Tray spacers  better (Autodesk Fusion 360 archive; units mm, degrees)
design "tray spacers"
Autodesk Fusion 360 part; units mm, degrees
(part 1 of 2)
sketch "Sketch1" plane through (0, 0, 0) normal (0, 1, 0) x (1, 0, 0)
  line L0 (21, -7) -> (-21, -7)
  line L1 (-21, -7) -> (-21, 7)
  line L2 (-21, 7) -> (21, 7)
  line L3 (21, 7) -> (21, -7)
  line L4 (21, -7) -> (-21, 7) construction
  line L5 (-21, -7) -> (21, 7) construction
  line L6 (7, -21) -> (-7, -21)
  line L7 (-7, -21) -> (-7, 21)
  line L8 (-7, 21) -> (7, 21)
  line L9 (7, 21) -> (7, -21)
  line L10 (7, -21) -> (-7, 21) construction
  line L11 (-7, -21) -> (7, 21) construction
  line L12 (23.58, 0) -> (93.58, 0)
  line L13 (93.58, 0) -> (93.58, 7)
  line L14 (93.58, 7) -> (23.58, 7)
  line L15 (23.58, 7) -> (23.58, 0)
  line L16 (58.58, 0) -> (51.58, 0)
  line L17 (51.58, 0) -> (51.58, 42)
  line L18 (51.58, 42) -> (58.58, 42)
  line L19 (58.58, 42) -> (58.58, 0)
  line L20 (58.58, 0) -> (65.58, 0)
  line L21 (65.58, 0) -> (65.58, 42)
  line L22 (65.58, 42) -> (58.58, 42)
  line L23 (58.58, 42) -> (58.58, 0)
  line L24 (101.6, 0) -> (143.6, 0)
  line L25 (143.6, 0) -> (143.6, 7)
  line L26 (143.6, 7) -> (101.6, 7)
  line L27 (101.6, 7) -> (101.6, 0)
  line L28 (143.6, 0) -> (136.6, 0)
  line L29 (136.6, 0) -> (136.6, 42)
  line L30 (136.6, 42) -> (143.6, 42)
  line L31 (143.6, 42) -> (143.6, 0)
  line L32 (-21, 57) -> (21, 57)
  line L33 (7, 71) -> (7, 29)
  line L34 (21, 57) -> (21, 43)
  line L35 (21, 43) -> (-21, 57) construction
  line L36 (-21, 43) -> (21, 57) construction
  line L37 (-7, 29) -> (7, 71) construction
  line L38 (21, 43) -> (-21, 43)
  line L39 (-21, 43) -> (-21, 57)
  line L40 (-7, 29) -> (-7, 71)
  line L41 (7, 29) -> (-7, 71) construction
  line L42 (-7, 71) -> (7, 71)
  line L43 (7, 29) -> (-7, 29)
  line L44 (93.58, 0) -> (23.58, 0)
  line L45 (23.58, 0) -> (23.58, -7)
  line L46 (23.58, -7) -> (93.58, -7)
  line L47 (93.58, -7) -> (93.58, 0)
  line L48 (101.6, 0) -> (150.6, 0)
  line L49 (150.6, 0) -> (150.6, -7)
  line L50 (150.6, -7) -> (101.6, -7)
  line L51 (101.6, -7) -> (101.6, 0)
  line L52 (150.6, -7) -> (143.6, -7)
  line L53 (143.6, -7) -> (143.6, 42)
  line L54 (143.6, 42) -> (150.6, 42)
  line L55 (150.6, 42) -> (150.6, -7)
  point P0 (0, 50)
  point P1 (0, 50)
  dimension "d1" = 42
  dimension "d2" = 14
  dimension "d3" = 14
  dimension "d4" = 42
  dimension "d5" = 70
  dimension "d6" = 7
  dimension "d7" = 7
  dimension "d8" = 42
  dimension "d9" = 7
  dimension "d10" = 42
  dimension "d11" = 42
  dimension "d12" = 7
  dimension "d13" = 7
  dimension "d14" = 42
  dimension "d15" = 42
  dimension "d16" = 14
  dimension "d17" = 14
  dimension "d18" = 42
  dimension "d25" = 7
  dimension "d26" = 49
  dimension "d27" = 7
  constraint horizontal L0
  constraint perpendicular L0 L1
  constraint parallel L0 L2
  constraint parallel L1 L3
  constraint coincident L4 origin
  constraint coincident L5 origin
  constraint horizontal L6
  constraint perpendicular L6 L7
  constraint parallel L6 L8
  constraint parallel L7 L9
  constraint coincident L10 origin
  constraint coincident L11 origin
  constraint horizontal L12
  constraint vertical L13
  constraint horizontal L14
  constraint vertical L15
  constraint horizontal L16
  constraint vertical L17
  constraint horizontal L18
  constraint vertical L19
  constraint midpoint L12 L16.start
  constraint horizontal L20
  constraint vertical L21
  constraint horizontal L22
  constraint vertical L23
  constraint horizontal L24
  constraint vertical L25
  constraint horizontal L26
  constraint vertical L27
  constraint horizontal L28
  constraint vertical L29
  constraint horizontal L30
  constraint vertical L31
  constraint horizontal L38
  constraint perpendicular L38 L39
  constraint parallel L32 L38
  constraint parallel L34 L39
  constraint coincident P1 L35
  constraint coincident P1 L36
  constraint horizontal L43
  constraint perpendicular L40 L43
  constraint parallel L42 L43
  constraint parallel L33 L40
  constraint coincident P1 L41
  constraint coincident P1 L37
  constraint coincident P1 P0
  constraint horizontal L44
  constraint vertical L45
  constraint horizontal L46
  constraint vertical L47
  constraint horizontal L48
  constraint vertical L49
  constraint horizontal L50
  constraint vertical L51
  constraint horizontal L52
  constraint vertical L53
  constraint horizontal L54
  constraint vertical L55
  measures "d1" distance of L1.end L2.end
  measures "d2" distance of L0.end L1.end
  measures "d3" distance of L7.end L8.end
  measures "d4" distance of L6.end L7.end
  measures "d5" distance of L12.start L12.end
  measures "d6" distance of L12.start L14.end
  measures "d7" distance of L16.start L16.end
  measures "d8" distance of L16.start L18.end
  measures "d9" distance of L16.start L20.end
  measures "d10" distance of L16.start L18.end
  measures "d11" distance of L24.start L24.end
  measures "d12" distance of L24.start L26.end
  measures "d13" distance of L24.end L28.end
  measures "d14" distance of L24.end L30.end
  measures "d15" distance of L32.start L32.end
  measures "d16" distance of L36.start L32.start
  measures "d17" distance of L33.start L40.end
  measures "d18" distance of L40.end L37.start
  measures "d25" distance of L12.end L46.end
  measures "d26" distance of L24.start L48.end
  measures "d27" distance of L24.start L50.end
extrude "Extrude1" add sketch "Sketch1" along normal blind 54 contours L0 L2 L3 L9 | L0 L6 L7 L9 | L0 L2 L7 L9 | L0 L1 L2 L7 | L2 L7 L8 L9 | L12 L14 L15 L17 L44 | L12 L16 L20 L44 L45 L46 L47 | L12 L14 L16 L17 L19 L23 L44 | L12 L14 L19 L20 L21 L23 L44 | L14 L17 L18 L19 L23 | L12 L13 L14 L21 L44 | L14 L19 L21 L22 L23 | L24 L26 L27 L29 L48 | L24 L28 L48 L50 L51 L53 | L24 L25 L26 L28 L29 L31 L48 L53 | L25 L31 L48 L53 L54 L55 | L48 L49 L50 L52 L53 L55 | L26 L29 L30 L31 L53 makes body 1 at (-16.3333, 0, -2.3333) makes body 2 at (46.9133, 18, 7) makes body 3 at (134.2667, 36, 7)
extrude "Extrude2" add sketch "Sketch1" along normal blind 12 separate body contours L32 L38 L39 L40 | L32 L33 L40 L42 | L32 L33 L38 L40 | L32 L33 L34 L38 | L33 L38 L40 L43 makes body 4
chamfer "Chamfer1" distance 6.99 angle 59 7 edges at (79.58, 54, -7) (65.58, 54, -24.5) (58.58, 54, -42) (51.58, 54, -24.5) (37.58, 54, -7) (136.6, 54, -24.5) (119.1, 54, -7) 2 faces at (-16.3333, 54, -2.3333) (-2.3333, 12, -33.6667) measured on face at (56.2467, 54, 2.3333) measured on face at (56.2467, 54, 2.3333) measured on face at (56.2467, 54, 2.3333) measured on face at (56.2467, 54, 2.3333) measured on face at (56.2467, 54, 2.3333) measured on face at (129.6, 54, 2.3333) measured on face at (129.6, 54, 2.3333) tangent chain off on bodies 1 2 3 4
extrude "Extrude3" add 2 faces at (131.93, 54, 4.6633) (58.5767, 54, 4.6633) along direction (0, 1, 0) blind 3 on bodies 2 3 bodies 3 2
extrude "Extrude4" cut 1 faces at (58.57, 55, -11.6767) along direction (1, 0, 0) blind 1 on bodies 2 bodies 2
sketch "Sketch2" plane through (0, 0, 7) normal (0, 0, 1) x (1, 0, 0)
  line L0 (23.58, 0) -> (93.58, 0)
  line L1 (93.58, 0) -> (93.58, 57)
  line L2 (93.58, 57) -> (23.58, 57)
  line L3 (23.58, 57) -> (23.58, 0)
  line L4 (93.58, 0) -> (58.58, 0)
  line L5 (58.58, 0) -> (58.58, 12)
  line L6 (58.58, 12) -> (93.58, 12)
  line L7 (93.58, 12) -> (93.58, 0)
  line L8 (58.58, 12) -> (58.58, 45)
  circle A0 centre (58.58, 12) radius 1.9
  circle A1 centre (58.58, 45) radius 1.9
  dimension "d32" = 35
  dimension "d33" = 12
  dimension "d34" = 33
  dimension "d35" = 3.8
  dimension "d36" = 3.8
  constraint horizontal L4
  constraint vertical L5
  constraint horizontal L6
  constraint vertical L7
  constraint coincident L0.end L1.start
  constraint perpendicular L6 L8
  constraint coincident L5.end L6.start
  constraint coincident L8.end A1.centre
  measures "d32" distance of L0.end L4.end
  measures "d33" distance of L0.end L6.end
  measures "d34" distance of L5.end L8.end
  measures "d35" diameter of A0
  measures "d36" diameter of A1
extrude "Extrude5" cut sketch "Sketch2" against normal blind 40 contours L5 L8 A0 | L5 L6 A0 | L6 L8 A0 | A1 bodies 2
sketch "Sketch3" plane through (0, 0, 0) normal (0, -1, 0) x (1, 0, 0)
  line L0 (23.58, -7) -> (51.58, -7)
  line L1 (51.58, -7) -> (51.58, -42)
  line L2 (51.58, -42) -> (65.58, -42)
  line L3 (65.58, -42) -> (65.58, -7)
  line L4 (65.58, -7) -> (93.58, -7)
  line L5 (93.58, -7) -> (93.58, 7)
  line L6 (93.58, 7) -> (23.58, 7)
  line L7 (23.58, 7) -> (23.58, -7)
  line L8 (23.58, 7) -> (30.58, 7)
  line L9 (30.58, 7) -> (30.58, 0)
  line L10 (30.58, 0) -> (23.58, 0)
  line L11 (23.58, 0) -> (23.58, 7)
  circle A0 centre (30.58, 0) radius 1.9
  line L12 (93.58, 7) -> (86.58, 7)
  line L13 (86.58, 7) -> (86.58, 0)
  line L14 (86.58, 0) -> (93.58, 0)
  line L15 (93.58, 0) -> (93.58, 7)
  circle A1 centre (86.58, 0) radius 1.9
  line L16 (51.58, -42) -> (58.58, -42)
  line L17 (58.58, -42) -> (58.58, -35)
  line L18 (58.58, -35) -> (51.58, -35)
  line L19 (51.58, -35) -> (51.58, -42)
  circle A2 centre (58.58, -35) radius 1.9
  dimension "d39" = 7
  dimension "d40" = 7
  dimension "d41" = 3.8
  dimension "d42" = 7
  dimension "d43" = 7
  dimension "d44" = 3.8
  dimension "d71" = 7
  dimension "d72" = 7
  dimension "d73" = 3.8
  constraint horizontal L8
  constraint vertical L9
  constraint horizontal L10
  constraint vertical L11
  constraint coincident L6.end L7.start
  constraint coincident L9.end L10.start
  constraint horizontal L12
  constraint vertical L13
  constraint horizontal L14
  constraint vertical L15
  constraint coincident L5.end L6.start
  constraint coincident L13.end L14.start
  constraint horizontal L16
  constraint vertical L17
  constraint horizontal L18
  constraint vertical L19
  constraint coincident L1.end L2.start
  constraint coincident L17.end L18.start
  measures "d39" distance of L6.end L8.end
  measures "d40" distance of L6.end L10.end
  measures "d41" diameter of A0
  measures "d42" distance of L5.end L12.end
  measures "d43" distance of L5.end L14.end
  measures "d44" diameter of A1
  measures "d71" distance of L1.end L16.end
  measures "d72" distance of L1.end L18.end
  measures "d73" diameter of A2
sketch "Sketch4" plane through (0, 0, 0) normal (0, -1, 0) x (1, 0, 0)
  line L0 (101.6, -7) -> (136.6, -7)
  line L1 (136.6, -7) -> (136.6, -42)
  line L2 (136.6, -42) -> (150.6, -42)
  line L3 (150.6, -42) -> (150.6, 7)
  line L4 (150.6, 7) -> (101.6, 7)
  line L5 (101.6, 7) -> (101.6, -7)
  line L6 (101.6, 7) -> (108.6, 7)
  line L7 (108.6, 7) -> (108.6, 0)
  line L8 (108.6, 0) -> (101.6, 0)
  line L9 (101.6, 0) -> (101.6, 7)
  circle A0 centre (108.6, 0) radius 1.9
  line L10 (150.6, -42) -> (143.6, -42)
  line L11 (143.6, -42) -> (143.6, -35)
  line L12 (143.6, -35) -> (150.6, -35)
  line L13 (150.6, -35) -> (150.6, -42)
  circle A1 centre (143.6, -35) radius 1.75
  dimension "d45" = 7
  dimension "d46" = 7
  dimension "d47" = 3.8
  dimension "d48" = 7
  dimension "d49" = 7
  dimension "d54" = 3.5
  constraint horizontal L6
  constraint vertical L7
  constraint horizontal L8
  constraint vertical L9
  constraint coincident L4.end L5.start
  constraint coincident L7.end L8.start
  constraint horizontal L10
  constraint vertical L11
  constraint horizontal L12
  constraint vertical L13
  constraint coincident L2.end L3.start
  constraint coincident L11.end L12.start
  measures "d45" distance of L4.end L6.end
  measures "d46" distance of L4.end L8.end
  measures "d47" diameter of A0
  measures "d48" distance of L2.end L10.end
  measures "d49" distance of L2.end L12.end
  measures "d54" diameter of A1
sketch "Sketch5" plane through (0, 0, 0) normal (0, -1, 0) x (1, 0, 0)
  line L0 (-7, -21) -> (7, -21)
  line L1 (7, -21) -> (7, -7)
  line L2 (7, -7) -> (21, -7)
  line L3 (21, -7) -> (21, 7)
  line L4 (21, 7) -> (7, 7)
  line L5 (7, 7) -> (7, 21)
  line L6 (7, 21) -> (-7, 21)
  line L7 (-7, 21) -> (-7, 7)
  line L8 (-7, 7) -> (-21, 7)
  line L9 (-21, 7) -> (-21, -7)
  line L10 (-21, -7) -> (-7, -7)
  line L11 (-7, -7) -> (-7, -21)
  line L12 (-7, 7) -> (0, 7)
  line L13 (0, 7) -> (0, 0)
  line L14 (0, 0) -> (-7, 0)
  line L15 (-7, 0) -> (-7, 7)
  circle A0 centre (0, 0) radius 1.9
  dimension "d51" = 3.8
  constraint horizontal L12
  constraint vertical L13
  constraint horizontal L14
  constraint vertical L15
  constraint coincident L7.end L8.start
  constraint coincident L13.end L14.start
  measures "d51" diameter of A0
extrude "Extrude6" cut sketch "Sketch5" sketch "Sketch3" sketch "Sketch4" against normal blind 40 contours L13 L14 A0 | L13 L14 A0 of sketch 2 contours L9 L10 A0 | L9 L10 A0 | L17 L18 A2 | L17 L18 A2 | L13 L14 A1 | L13 L14 A1 of sketch 3 contours L7 L8 A0 | L7 L8 A0 | L11 L12 A1 | L11 L12 A1 bodies 1 2 3
sketch "Sketch6" plane through (0, 0, 7) normal (0, 0, 1) x (1, 0, 0)
  line L0 (101.6, 0) -> (150.6, 0)
  line L1 (150.6, 0) -> (150.6, 57)
  line L2 (150.6, 57) -> (101.6, 57)
  line L3 (101.6, 57) -> (101.6, 0)
  line L4 (150.6, 57) -> (143.6, 57)
  line L5 (143.6, 57) -> (143.6, 47)
  line L6 (143.6, 47) -> (150.6, 47)
  line L7 (150.6, 47) -> (150.6, 57)
  line L8 (150.6, 0) -> (143.6, 0)
  line L9 (143.6, 0) -> (143.6, 14)
  line L10 (143.6, 14) -> (150.6, 14)
  line L11 (150.6, 14) -> (150.6, 0)
  circle A0 centre (143.6, 14) radius 1.9
  circle A1 centre (143.6, 47) radius 1.9
  dimension "d55" = 7
  dimension "d56" = 10
  dimension "d57" = 7
  dimension "d58" = 14
  dimension "d59" = 3.8
  dimension "d60" = 3.8
  constraint horizontal L4
  constraint vertical L5
  constraint horizontal L6
  constraint vertical L7
  constraint coincident L1.end L2.start
  constraint horizontal L8
  constraint vertical L9
  constraint horizontal L10
  constraint vertical L11
  constraint coincident L0.end L1.start
  constraint coincident L9.end L10.start
  constraint coincident L5.end L6.start
  measures "d55" distance of L1.end L4.end
  measures "d56" distance of L1.end L6.end
  measures "d57" distance of L0.end L8.end
  measures "d58" distance of L0.end L10.end
  measures "d59" diameter of A0
  measures "d60" diameter of A1
extrude "Extrude7" cut sketch "Sketch6" against normal blind 40 contours L9 L10 A0 | L9 L10 A0 | L5 L6 A1 | L5 L6 A1 bodies 3
sketch "Sketch7" plane through (150.6, 0, 0) normal (1, 0, 0) x (0, 0, -1)
  line L0 (-7, 0) -> (42, 0)
  line L1 (42, 0) -> (42, 57)
  line L2 (42, 57) -> (-7, 57)
  line L3 (-7, 57) -> (-7, 0)
  line L4 (-7, 57) -> (0, 57)
  line L5 (0, 57) -> (0, 43)
  line L6 (0, 43) -> (-7, 43)
  line L7 (-7, 43) -> (-7, 57)
  line L8 (-7, 0) -> (0, 0)
  line L9 (0, 0) -> (0, 10)
  line L10 (0, 10) -> (-7, 10)
  line L11 (-7, 10) -> (-7, 0)
  circle A0 centre (0, 10) radius 1.9
  circle A1 centre (0, 43) radius 1.9
  dimension "d63" = 7
  dimension "d64" = 14
  dimension "d65" = 7
  dimension "d66" = 10
  dimension "d67" = 3.8
  dimension "d68" = 3.8
  constraint horizontal L4
  constraint vertical L5
  constraint horizontal L6
  constraint vertical L7
  constraint coincident L2.end L3.start
  constraint horizontal L8
  constraint vertical L9
  constraint horizontal L10
  constraint vertical L11
  constraint coincident L0.start L3.end
  constraint coincident L9.end L10.start
  constraint coincident L5.end L6.start
  measures "d63" distance of L2.end L4.end
  measures "d64" distance of L2.end L6.end
  measures "d65" distance of L0.start L8.end
  measures "d66" distance of L0.start L10.end
  measures "d67" diameter of A0
  measures "d68" diameter of A1
extrude "Extrude8" cut sketch "Sketch7" against normal blind 40 contours L9 L10 A0 | L9 L10 A0 | L5 L6 A1 | L5 L6 A1 bodies 3
move_body "Move29" bodies 3 to x (1, 0, 0) y (0, 1, 0) z (0, 0, 1) at (13.98, 0, 0)
copy_body "CopyPasteBodies17" bodies 2 makes body 5
move_body "Move30" bodies 5 to x (1, 0, 0) y (0, 1, 0) z (0, 0, 1) at (-99, 0, 0)
copy_body "CopyPasteBodies18" bodies 2 5 makes body 6 makes body 7
move_body "Move31" bodies 6 7 to x (1, 0, 0) y (0, 1, 0) z (0, 0, 1) at (-198, 0, 0)
copy_body "CopyPasteBodies21" bodies 7 makes body 8
move_body "Move34" bodies 8 to x (1, 0, 0) y (0, 1, 0) z (0, 0, 1) at (-99, 0, 0)
copy_body "CopyPasteBodies20" bodies 3 makes body 9
move_body "Move33" bodies 9 to x (0, 0, 1) y (0, 1, 0) z (-1, 0, 0) at (-436.42, 0, -157.58)
copy_body "CopyPasteBodies23" bodies 2 makes body 10
move_body "Move36" bodies 10 to x (0, 0, -1) y (0, 1, 0) z (1, 0, 0) at (157.58, 0, -82.42)
copy_body "CopyPasteBodies24" bodies 10 makes body 11
move_body "Move37" bodies 11 to x (1, 0, 0) y (0, 1, 0) z (0, 0, 1) at (0, 0, -141)
copy_body "CopyPasteBodies25" bodies 11 makes body 12
move_body "Move38" bodies 12 to x (1, 0, 0) y (0, 1, 0) z (0, 0, 1) at (0, 0, -141)
copy_body "CopyPasteBodies26" bodies 2 3 5 6 7 8 9 10 11 12 makes body 13 makes body 14 makes body 15 makes body 16 makes body 17 makes body 18 makes body 19 makes body 20 makes body 21 makes body 22
move_body "Move39" bodies 13 14 15 16 17 18 19 20 21 22 to x (-1, 0, 0) y (0, 1, 0) z (0, 0, -1) at (-278.84, 0, -564)
move_body "Move40" bodies 1 to x (1, 0, 0) y (0, 1, 0) z (0, 0, 1) at (59, 0, -61)
move_body "Move41" bodies 1 to x (1, 0, 0) y (0, 1, 0) z (0, 0, 1) at (-0.42, 0, -80)
move_body "Move42" bodies 4 to x (1, 0, 0) y (0, 1, 0) z (0, 0, 1) at (58.58, 0, -91)
move_body "Move43" bodies 4 to x (1, 0, 0) y (0, 1, 0) z (0, 0, 1) at (0, 0, -141)
copy_body "CopyPasteBodies27" bodies 1 makes body 23
move_body "Move44" bodies 23 to x (1, 0, 0) y (0, 1, 0) z (0, 0, 1) at (0, 0, -282)
copy_body "CopyPasteBodies29" bodies 1 4 23 makes body 24 makes body 25 makes body 26
move_body "Move46" bodies 24 25 26 to x (1, 0, 0) y (0, 1, 0) z (0, 0, 1) at (-198, 0, 0)
copy_body "CopyPasteBodies30" bodies 24 26 25 makes body 27 makes body 28 makes body 29
move_body "Move47" bodies 27 28 29 to x (1, 0, 0) y (0, 1, 0) z (0, 0, 1) at (-198, 0, 0)
copy_body "CopyPasteBodies31" bodies 4 makes body 30
move_body "Move48" bodies 30 to x (1, 0, 0) y (0, 1, 0) z (0, 0, 1) at (-99, 0, 141)
copy_body "CopyPasteBodies32" bodies 30 makes body 31
move_body "Move49" bodies 31 to x (1, 0, 0) y (0, 1, 0) z (0, 0, 1) at (0, 0, -282)
copy_body "CopyPasteBodies33" bodies 1 makes body 32
move_body "Move50" bodies 32 to x (1, 0, 0) y (0, 1, 0) z (0, 0, 1) at (-99, 0, -141)
copy_body "CopyPasteBodies34" bodies 30 31 32 makes body 33 makes body 34 makes body 35
move_body "Move51" bodies 33 34 35 to x (1, 0, 0) y (0, 1, 0) z (0, 0, 1) at (-198, 0, 0)
sketch "Sketch8" plane through (0, 0, 0) normal (0, -1, 0) x (1, 0, 0)
  circle A0 centre (-436.42, -35) radius 1.9
  circle A1 centre (-401.42, 0) radius 1.75
  line L0 (-429.42, -42) -> (-429.42, -7)
  line L1 (-429.42, -7) -> (-394.42, -7)
  line L2 (-394.42, -7) -> (-394.42, 7)
  line L3 (-394.42, 7) -> (-443.42, 7)
  line L4 (-443.42, 7) -> (-443.42, -42)
  line L5 (-443.42, -42) -> (-429.42, -42)
  line L6 (-443.42, 7) -> (164.58, 7)
  line L7 (164.58, 7) -> (164.58, -571)
  line L8 (164.58, -571) -> (-443.42, -571)
  line L9 (-443.42, -571) -> (-443.42, 7)
  line L10 (164.58, -571) -> (169.58, -571)
  line L11 (169.58, -571) -> (169.58, -576)
  line L12 (169.58, -576) -> (164.58, -576)
  line L13 (164.58, -576) -> (164.58, -571)
  line L14 (-443.42, 7) -> (-448.42, 7)
  line L15 (-448.42, 7) -> (-448.42, 12)
  line L16 (-448.42, 12) -> (-443.42, 12)
  line L17 (-443.42, 12) -> (-443.42, 7)
  line L18 (-448.42, 12) -> (169.58, 12)
  line L19 (169.58, 12) -> (169.58, -576)
  line L20 (169.58, -576) -> (-448.42, -576)
  line L21 (-448.42, -576) -> (-448.42, 12)
  dimension "d74" = 608
  dimension "d75" = 578
  dimension "d76" = 5
  dimension "d77" = 5
  dimension "d78" = 5
  dimension "d79" = 5
  constraint horizontal L6
  constraint vertical L7
  constraint horizontal L8
  constraint vertical L9
  constraint coincident L3.end L4.start
  constraint horizontal L10
  constraint vertical L11
  constraint horizontal L12
  constraint vertical L13
  constraint horizontal L14
  constraint vertical L15
  constraint horizontal L16
  constraint vertical L17
  constraint horizontal L18
  constraint vertical L19
  constraint horizontal L20
  constraint vertical L21
  measures "d74" distance of L3.end L6.end
  measures "d75" distance of L3.end L8.end
  measures "d76" distance of L7.end L10.end
  measures "d77" distance of L7.end L12.end
  measures "d78" distance of L3.end L14.end
  measures "d79" distance of L3.end L16.end
extrude "Extrude9" add sketch "Sketch8" along normal blind 5 contours A0 | A1 | L0 L1 L2 L3 L4 L5 L6 L9 | L0 L1 L2 L5 L6 L7 L8 L9 bodies 1 2 3 4 5 6 7 8 9 10 11 12 13 14 15 16 17 18 19 20 21 22 23 24 25 26 27 28 29 30 31 32 33 34 35
extrude "Extrude10" add sketch "Sketch8" along normal blind -57 and the other way blind -5 separate body contours L4 L8 L9 L13 L14 L20 L21 | L3 L6 L7 L10 L17 L18 L19 | L14 L15 L16 L17 L18 L21 | L10 L11 L12 L13 L19 L20 makes body 36
sketch "Sketch9" plane through (0, 0, 0) normal (0, 1, 0) x (-1, 0, 0)
  line L0 (429.42, -106) -> (443.42, -106)
  line L1 (443.42, -106) -> (443.42, -42)
  line L2 (443.42, -42) -> (429.42, -42)
  line L3 (429.42, -42) -> (429.42, -7)
  line L4 (429.42, -7) -> (394.42, -7)
  line L5 (394.42, -7) -> (394.42, 7)
  line L6 (394.42, 7) -> (372.42, 7)
  line L7 (372.42, 7) -> (372.42, -7)
  line L8 (372.42, -7) -> (344.42, -7)
  line L9 (344.42, -7) -> (344.42, -42)
  line L10 (344.42, -42) -> (330.42, -42)
  line L11 (330.42, -42) -> (330.42, -7)
  line L12 (330.42, -7) -> (302.42, -7)
  line L13 (302.42, -7) -> (302.42, 7)
  line L14 (302.42, 7) -> (273.42, 7)
  line L15 (273.42, 7) -> (273.42, -7)
  line L16 (273.42, -7) -> (245.42, -7)
  line L17 (245.42, -7) -> (245.42, -42)
  line L18 (245.42, -42) -> (231.42, -42)
  line L19 (231.42, -42) -> (231.42, -7)
  line L20 (231.42, -7) -> (203.42, -7)
  line L21 (203.42, -7) -> (203.42, 7)
  line L22 (203.42, 7) -> (174.42, 7)
  line L23 (174.42, 7) -> (174.42, -7)
  line L24 (174.42, -7) -> (146.42, -7)
  line L25 (146.42, -7) -> (146.42, -42)
  line L26 (146.42, -42) -> (132.42, -42)
  line L27 (132.42, -42) -> (132.42, -7)
  line L28 (132.42, -7) -> (104.42, -7)
  line L29 (104.42, -7) -> (104.42, 7)
  line L30 (104.42, 7) -> (75.42, 7)
  line L31 (75.42, 7) -> (75.42, -7)
  line L32 (75.42, -7) -> (47.42, -7)
  line L33 (47.42, -7) -> (47.42, -42)
  line L34 (47.42, -42) -> (33.42, -42)
  line L35 (33.42, -42) -> (33.42, -7)
  line L36 (33.42, -7) -> (5.42, -7)
  line L37 (5.42, -7) -> (5.42, 7)
  line L38 (5.42, 7) -> (-23.58, 7)
  line L39 (-23.58, 7) -> (-23.58, -7)
  line L40 (-23.58, -7) -> (-51.58, -7)
  line L41 (-51.58, -7) -> (-51.58, -42)
  line L42 (-51.58, -42) -> (-65.58, -42)
  line L43 (-65.58, -42) -> (-65.58, -7)
  line L44 (-65.58, -7) -> (-93.58, -7)
  line L45 (-93.58, -7) -> (-93.58, 7)
  line L46 (-93.58, 7) -> (-115.58, 7)
  line L47 (-115.58, 7) -> (-115.58, -7)
  line L48 (-115.58, -7) -> (-150.58, -7)
  line L49 (-150.58, -7) -> (-150.58, -42)
  line L50 (-150.58, -42) -> (-164.58, -42)
  line L51 (-164.58, -42) -> (-164.58, -106)
  line L52 (-164.58, -106) -> (-150.58, -106)
  line L53 (-150.58, -106) -> (-150.58, -134)
  line L54 (-150.58, -134) -> (-115.58, -134)
  line L55 (-115.58, -134) -> (-115.58, -148)
  line L56 (-115.58, -148) -> (-150.58, -148)
  line L57 (-150.58, -148) -> (-150.58, -176)
  line L58 (-150.58, -176) -> (-164.58, -176)
  line L59 (-164.58, -176) -> (-164.58, -247)
  line L60 (-164.58, -247) -> (-150.58, -247)
  line L61 (-150.58, -247) -> (-150.58, -275)
  line L62 (-150.58, -275) -> (-115.58, -275)
  line L63 (-115.58, -275) -> (-115.58, -289)
  line L64 (-115.58, -289) -> (-150.58, -289)
  line L65 (-150.58, -289) -> (-150.58, -317)
  line L66 (-150.58, -317) -> (-164.58, -317)
  line L67 (-164.58, -317) -> (-164.58, -388)
  line L68 (-164.58, -388) -> (-150.58, -388)
  line L69 (-150.58, -388) -> (-150.58, -416)
  line L70 (-150.58, -416) -> (-115.58, -416)
  line L71 (-115.58, -416) -> (-115.58, -430)
  line L72 (-115.58, -430) -> (-150.58, -430)
  line L73 (-150.58, -430) -> (-150.58, -458)
  line L74 (-150.58, -458) -> (-164.58, -458)
  line L75 (-164.58, -458) -> (-164.58, -522)
  line L76 (-164.58, -522) -> (-150.58, -522)
  line L77 (-150.58, -522) -> (-150.58, -557)
  line L78 (-150.58, -557) -> (-115.58, -557)
  line L79 (-115.58, -557) -> (-115.58, -571)
  line L80 (-115.58, -571) -> (-93.58, -571)
  line L81 (-93.58, -571) -> (-93.58, -557)
  line L82 (-93.58, -557) -> (-65.58, -557)
  line L83 (-65.58, -557) -> (-65.58, -522)
  line L84 (-65.58, -522) -> (-51.58, -522)
  line L85 (-51.58, -522) -> (-51.58, -557)
  line L86 (-51.58, -557) -> (-23.58, -557)
  line L87 (-23.58, -557) -> (-23.58, -571)
  line L88 (-23.58, -571) -> (5.42, -571)
  line L89 (5.42, -571) -> (5.42, -557)
  line L90 (5.42, -557) -> (33.42, -557)
  line L91 (33.42, -557) -> (33.42, -522)
  line L92 (33.42, -522) -> (47.42, -522)
  line L93 (47.42, -522) -> (47.42, -557)
  line L94 (47.42, -557) -> (75.42, -557)
  line L95 (75.42, -557) -> (75.42, -571)
  line L96 (75.42, -571) -> (104.42, -571)
  line L97 (104.42, -571) -> (104.42, -557)
  line L98 (104.42, -557) -> (132.42, -557)
  line L99 (132.42, -557) -> (132.42, -522)
  line L100 (132.42, -522) -> (146.42, -522)
  line L101 (146.42, -522) -> (146.42, -557)
  line L102 (146.42, -557) -> (174.42, -557)
  line L103 (174.42, -557) -> (174.42, -571)
  line L104 (174.42, -571) -> (203.42, -571)
  line L105 (203.42, -571) -> (203.42, -557)
  line L106 (203.42, -557) -> (231.42, -557)
  line L107 (231.42, -557) -> (231.42, -522)
  line L108 (231.42, -522) -> (245.42, -522)
  line L109 (245.42, -522) -> (245.42, -557)
  line L110 (245.42, -557) -> (273.42, -557)
  line L111 (273.42, -557) -> (273.42, -571)
  line L112 (273.42, -571) -> (302.42, -571)
  line L113 (302.42, -571) -> (302.42, -557)
  line L114 (302.42, -557) -> (330.42, -557)
  line L115 (330.42, -557) -> (330.42, -522)
  line L116 (330.42, -522) -> (344.42, -522)
  line L117 (344.42, -522) -> (344.42, -557)
  line L118 (344.42, -557) -> (372.42, -557)
  line L119 (372.42, -557) -> (372.42, -571)
  line L120 (372.42, -571) -> (394.42, -571)
  line L121 (394.42, -571) -> (394.42, -557)
  line L122 (394.42, -557) -> (429.42, -557)
  line L123 (429.42, -557) -> (429.42, -522)
  line L124 (429.42, -522) -> (443.42, -522)
  line L125 (443.42, -522) -> (443.42, -458)
  line L126 (443.42, -458) -> (429.42, -458)
  line L127 (429.42, -458) -> (429.42, -430)
  line L128 (429.42, -430) -> (394.42, -430)
  line L129 (394.42, -430) -> (394.42, -416)
  line L130 (394.42, -416) -> (429.42, -416)
  line L131 (429.42, -416) -> (429.42, -388)
  line L132 (429.42, -388) -> (443.42, -388)
  line L133 (443.42, -388) -> (443.42, -317)
  line L134 (443.42, -317) -> (429.42, -317)
  line L135 (429.42, -317) -> (429.42, -289)
  line L136 (429.42, -289) -> (394.42, -289)
  line L137 (394.42, -289) -> (394.42, -275)
  line L138 (394.42, -275) -> (429.42, -275)
  line L139 (429.42, -275) -> (429.42, -247)
  line L140 (429.42, -247) -> (443.42, -247)
  line L141 (443.42, -247) -> (443.42, -176)
  line L142 (443.42, -176) -> (429.42, -176)
  line L143 (429.42, -176) -> (429.42, -148)
  line L144 (429.42, -148) -> (394.42, -148)
  line L145 (394.42, -148) -> (394.42, -134)
  line L146 (394.42, -134) -> (429.42, -134)
  line L147 (429.42, -134) -> (429.42, -106)
  line L148 (231.42, -303) -> (231.42, -289)
  line L149 (231.42, -289) -> (217.42, -289)
  line L150 (217.42, -289) -> (217.42, -275)
  line L151 (217.42, -275) -> (231.42, -275)
  line L152 (231.42, -275) -> (231.42, -261)
  line L153 (231.42, -261) -> (245.42, -261)
  line L154 (245.42, -261) -> (245.42, -275)
  line L155 (245.42, -275) -> (259.42, -275)
  line L156 (259.42, -275) -> (259.42, -289)
  line L157 (259.42, -289) -> (245.42, -289)
  line L158 (245.42, -289) -> (245.42, -303)
  line L159 (245.42, -303) -> (231.42, -303)
  line L160 (231.42, -120) -> (245.42, -120)
  line L161 (245.42, -120) -> (245.42, -134)
  line L162 (245.42, -134) -> (259.42, -134)
  line L163 (259.42, -134) -> (259.42, -148)
  line L164 (259.42, -148) -> (245.42, -148)
  line L165 (245.42, -148) -> (245.42, -162)
  line L166 (245.42, -162) -> (231.42, -162)
  line L167 (231.42, -162) -> (231.42, -148)
  line L168 (231.42, -148) -> (217.42, -148)
  line L169 (217.42, -148) -> (217.42, -134)
  line L170 (217.42, -134) -> (231.42, -134)
  line L171 (231.42, -134) -> (231.42, -120)
  line L172 (33.42, -402) -> (47.42, -402)
  line L173 (47.42, -402) -> (47.42, -416)
  line L174 (47.42, -416) -> (61.42, -416)
  line L175 (61.42, -416) -> (61.42, -430)
  line L176 (61.42, -430) -> (47.42, -430)
  line L177 (47.42, -430) -> (47.42, -444)
  line L178 (47.42, -444) -> (33.42, -444)
  line L179 (33.42, -444) -> (33.42, -430)
  line L180 (33.42, -430) -> (19.42, -430)
  line L181 (19.42, -430) -> (19.42, -416)
  line L182 (19.42, -416) -> (33.42, -416)
  line L183 (33.42, -416) -> (33.42, -402)
  line L184 (330.42, -261) -> (344.42, -261)
  line L185 (344.42, -261) -> (344.42, -275)
  line L186 (344.42, -275) -> (358.42, -275)
  line L187 (358.42, -275) -> (358.42, -289)
  line L188 (358.42, -289) -> (344.42, -289)
  line L189 (344.42, -289) -> (344.42, -303)
  line L190 (344.42, -303) -> (330.42, -303)
  line L191 (330.42, -303) -> (330.42, -289)
  line L192 (330.42, -289) -> (316.42, -289)
  line L193 (316.42, -289) -> (316.42, -275)
  line L194 (316.42, -275) -> (330.42, -275)
  line L195 (330.42, -275) -> (330.42, -261)
  line L196 (330.42, -162) -> (330.42, -148)
  line L197 (330.42, -148) -> (316.42, -148)
  line L198 (316.42, -148) -> (316.42, -134)
  line L199 (316.42, -134) -> (330.42, -134)
  line L200 (330.42, -134) -> (330.42, -120)
  line L201 (330.42, -120) -> (344.42, -120)
  line L202 (344.42, -120) -> (344.42, -134)
  line L203 (344.42, -134) -> (358.42, -134)
  line L204 (358.42, -134) -> (358.42, -148)
  line L205 (358.42, -148) -> (344.42, -148)
  line L206 (344.42, -148) -> (344.42, -162)
  line L207 (344.42, -162) -> (330.42, -162)
  line L208 (132.42, -261) -> (146.42, -261)
  line L209 (146.42, -261) -> (146.42, -275)
  line L210 (146.42, -275) -> (160.42, -275)
  line L211 (160.42, -275) -> (160.42, -289)
  line L212 (160.42, -289) -> (146.42, -289)
  line L213 (146.42, -289) -> (146.42, -303)
  line L214 (146.42, -303) -> (132.42, -303)
  line L215 (132.42, -303) -> (132.42, -289)
  line L216 (132.42, -289) -> (118.42, -289)
  line L217 (118.42, -289) -> (118.42, -275)
  line L218 (118.42, -275) -> (132.42, -275)
  line L219 (132.42, -275) -> (132.42, -261)
  line L220 (-65.58, -444) -> (-65.58, -430)
  line L221 (-65.58, -430) -> (-79.58, -430)
  line L222 (-79.58, -430) -> (-79.58, -416)
  line L223 (-79.58, -416) -> (-65.58, -416)
  line L224 (-65.58, -416) -> (-65.58, -402)
  line L225 (-65.58, -402) -> (-51.58, -402)
  line L226 (-51.58, -402) -> (-51.58, -416)
  line L227 (-51.58, -416) -> (-37.58, -416)
  line L228 (-37.58, -416) -> (-37.58, -430)
  line L229 (-37.58, -430) -> (-51.58, -430)
  line L230 (-51.58, -430) -> (-51.58, -444)
  line L231 (-51.58, -444) -> (-65.58, -444)
  line L232 (-65.58, -162) -> (-65.58, -148)
  line L233 (-65.58, -148) -> (-79.58, -148)
  line L234 (-79.58, -148) -> (-79.58, -134)
  line L235 (-79.58, -134) -> (-65.58, -134)
  line L236 (-65.58, -134) -> (-65.58, -120)
  line L237 (-65.58, -120) -> (-51.58, -120)
  line L238 (-51.58, -120) -> (-51.58, -134)
  line L239 (-51.58, -134) -> (-37.58, -134)
  line L240 (-37.58, -134) -> (-37.58, -148)
  line L241 (-37.58, -148) -> (-51.58, -148)
  line L242 (-51.58, -148) -> (-51.58, -162)
  line L243 (-51.58, -162) -> (-65.58, -162)
  line L244 (-65.58, -261) -> (-51.58, -261)
  line L245 (-51.58, -261) -> (-51.58, -275)
  line L246 (-51.58, -275) -> (-37.58, -275)
  line L247 (-37.58, -275) -> (-37.58, -289)
  line L248 (-37.58, -289) -> (-51.58, -289)
  line L249 (-51.58, -289) -> (-51.58, -303)
  line L250 (-51.58, -303) -> (-65.58, -303)
  line L251 (-65.58, -303) -> (-65.58, -289)
  line L252 (-65.58, -289) -> (-79.58, -289)
  line L253 (-79.58, -289) -> (-79.58, -275)
  line L254 (-79.58, -275) -> (-65.58, -275)
  line L255 (-65.58, -275) -> (-65.58, -261)
  line L256 (132.42, -162) -> (132.42, -148)
  line L257 (132.42, -148) -> (118.42, -148)
  line L258 (118.42, -148) -> (118.42, -134)
  line L259 (118.42, -134) -> (132.42, -134)
  line L260 (132.42, -134) -> (132.42, -120)
  line L261 (132.42, -120) -> (146.42, -120)
  line L262 (146.42, -120) -> (146.42, -134)
  line L263 (146.42, -134) -> (160.42, -134)
  line L264 (160.42, -134) -> (160.42, -148)
  line L265 (160.42, -148) -> (146.42, -148)
  line L266 (146.42, -148) -> (146.42, -162)
  line L267 (146.42, -162) -> (132.42, -162)
  line L268 (132.42, -444) -> (132.42, -430)
  line L269 (132.42, -430) -> (118.42, -430)
  line L270 (118.42, -430) -> (118.42, -416)
  line L271 (118.42, -416) -> (132.42, -416)
  line L272 (132.42, -416) -> (132.42, -402)
  line L273 (132.42, -402) -> (146.42, -402)
  line L274 (146.42, -402) -> (146.42, -416)
  line L275 (146.42, -416) -> (160.42, -416)
  line L276 (160.42, -416) -> (160.42, -430)
  line L277 (160.42, -430) -> (146.42, -430)
  line L278 (146.42, -430) -> (146.42, -444)
  line L279 (146.42, -444) -> (132.42, -444)
  line L280 (330.42, -444) -> (330.42, -430)
  line L281 (330.42, -430) -> (316.42, -430)
  line L282 (316.42, -430) -> (316.42, -416)
  line L283 (316.42, -416) -> (330.42, -416)
  line L284 (330.42, -416) -> (330.42, -402)
  line L285 (330.42, -402) -> (344.42, -402)
  line L286 (344.42, -402) -> (344.42, -416)
  line L287 (344.42, -416) -> (358.42, -416)
  line L288 (358.42, -416) -> (358.42, -430)
  line L289 (358.42, -430) -> (344.42, -430)
  line L290 (344.42, -430) -> (344.42, -444)
  line L291 (344.42, -444) -> (330.42, -444)
  line L292 (33.42, -120) -> (47.42, -120)
  line L293 (47.42, -120) -> (47.42, -134)
  line L294 (47.42, -134) -> (61.42, -134)
  line L295 (61.42, -134) -> (61.42, -148)
  line L296 (61.42, -148) -> (47.42, -148)
  line L297 (47.42, -148) -> (47.42, -162)
  line L298 (47.42, -162) -> (33.42, -162)
  line L299 (33.42, -162) -> (33.42, -148)
  line L300 (33.42, -148) -> (19.42, -148)
  line L301 (19.42, -148) -> (19.42, -134)
  line L302 (19.42, -134) -> (33.42, -134)
  line L303 (33.42, -134) -> (33.42, -120)
  line L304 (33.42, -303) -> (33.42, -289)
  line L305 (33.42, -289) -> (19.42, -289)
  line L306 (19.42, -289) -> (19.42, -275)
  line L307 (19.42, -275) -> (33.42, -275)
  line L308 (33.42, -275) -> (33.42, -261)
  line L309 (33.42, -261) -> (47.42, -261)
  line L310 (47.42, -261) -> (47.42, -275)
  line L311 (47.42, -275) -> (61.42, -275)
  line L312 (61.42, -275) -> (61.42, -289)
  line L313 (61.42, -289) -> (47.42, -289)
  line L314 (47.42, -289) -> (47.42, -303)
  line L315 (47.42, -303) -> (33.42, -303)
  line L316 (231.42, -402) -> (245.42, -402)
  line L317 (245.42, -402) -> (245.42, -416)
  line L318 (245.42, -416) -> (259.42, -416)
  line L319 (259.42, -416) -> (259.42, -430)
  line L320 (259.42, -430) -> (245.42, -430)
  line L321 (245.42, -430) -> (245.42, -444)
  line L322 (245.42, -444) -> (231.42, -444)
  line L323 (231.42, -444) -> (231.42, -430)
  line L324 (231.42, -430) -> (217.42, -430)
  line L325 (217.42, -430) -> (217.42, -416)
  line L326 (217.42, -416) -> (231.42, -416)
  line L327 (231.42, -416) -> (231.42, -402)
  line L328 (33.42, -275) -> (-51.58, -275)
  line L329 (-51.58, -275) -> (-51.58, -148)
  line L330 (-51.58, -148) -> (33.42, -148)
  line L331 (33.42, -148) -> (33.42, -275)
  line L332 (33.42, -148) -> (27.22, -148)
  line L333 (27.22, -148) -> (27.22, -158)
  line L334 (27.22, -158) -> (33.42, -158)
  line L335 (33.42, -158) -> (33.42, -148)
  line L336 (27.22, -158) -> (-46.58, -158)
  line L337 (-46.58, -158) -> (-46.58, -269.2)
  line L338 (-46.58, -269.2) -> (27.22, -269.2)
  line L339 (27.22, -269.2) -> (27.22, -158)
  line L340 (27.22, -158) -> (9.52, -158)
  line L341 (9.52, -158) -> (9.52, -175.7)
  line L342 (9.52, -175.7) -> (27.22, -175.7)
  line L343 (27.22, -175.7) -> (27.22, -158)
  line L344 (-46.58, -158) -> (-28.88, -158)
  line L345 (-28.88, -158) -> (-28.88, -175.7)
  line L346 (-28.88, -175.7) -> (-46.58, -175.7)
  line L347 (-46.58, -175.7) -> (-46.58, -158)
  line L348 (-46.58, -269.2) -> (-28.88, -269.2)
  line L349 (-28.88, -269.2) -> (-28.88, -251.5)
  line L350 (-28.88, -251.5) -> (-46.58, -251.5)
  line L351 (-46.58, -251.5) -> (-46.58, -269.2)
  line L352 (27.22, -269.2) -> (9.52, -269.2)
  line L353 (9.52, -269.2) -> (9.52, -251.5)
  line L354 (9.52, -251.5) -> (27.22, -251.5)
  line L355 (27.22, -251.5) -> (27.22, -269.2)
  line L356 (9.52, -251.5) -> (8.52, -251.5)
  line L357 (8.52, -251.5) -> (8.52, -250.5)
  line L358 (8.52, -250.5) -> (9.52, -250.5)
  line L359 (9.52, -250.5) -> (9.52, -251.5)
  line L360 (8.52, -250.5) -> (-9.18, -250.5)
  line L361 (-9.18, -250.5) -> (-9.18, -232.8)
  line L362 (-9.18, -232.8) -> (8.52, -232.8)
  line L363 (8.52, -232.8) -> (8.52, -250.5)
  line L364 (8.52, -232.8) -> (9.52, -232.8)
  line L365 (9.52, -232.8) -> (9.52, -231.8)
  line L366 (9.52, -231.8) -> (8.52, -231.8)
  line L367 (8.52, -231.8) -> (8.52, -232.8)
  line L368 (9.52, -231.8) -> (27.22, -231.8)
  line L369 (27.22, -231.8) -> (27.22, -214.1)
  line L370 (27.22, -214.1) -> (9.52, -214.1)
  line L371 (9.52, -214.1) -> (9.52, -231.8)
  line L372 (9.52, -214.1) -> (8.52, -214.1)
  line L373 (8.52, -214.1) -> (8.52, -213.1)
  line L374 (8.52, -213.1) -> (9.52, -213.1)
  line L375 (9.52, -213.1) -> (9.52, -214.1)
  line L376 (8.52, -213.1) -> (-9.18, -213.1)
  line L377 (-9.18, -213.1) -> (-9.18, -195.4)
  line L378 (-9.18, -195.4) -> (8.52, -195.4)
  line L379 (8.52, -195.4) -> (8.52, -213.1)
  line L380 (8.52, -195.4) -> (9.52, -195.4)
  line L381 (9.52, -195.4) -> (9.52, -194.4)
  line L382 (9.52, -194.4) -> (8.52, -194.4)
  line L383 (8.52, -194.4) -> (8.52, -195.4)
  line L384 (9.52, -194.4) -> (27.22, -194.4)
  line L385 (27.22, -194.4) -> (27.22, -176.7)
  line L386 (27.22, -176.7) -> (9.52, -176.7)
  line L387 (9.52, -176.7) -> (9.52, -194.4)
  line L388 (9.52, -175.7) -> (8.52, -175.7)
  line L389 (8.52, -175.7) -> (8.52, -176.7)
  line L390 (8.52, -176.7) -> (9.52, -176.7)
  line L391 (9.52, -176.7) -> (9.52, -175.7)
  line L392 (8.52, -176.7) -> (-9.18, -176.7)
  line L393 (-9.18, -176.7) -> (-9.18, -194.4)
  line L394 (-9.18, -194.4) -> (8.52, -194.4)
  line L395 (8.52, -194.4) -> (8.52, -176.7)
  line L396 (-9.18, -176.7) -> (-10.18, -176.7)
  line L397 (-10.18, -176.7) -> (-10.18, -175.7)
  line L398 (-10.18, -175.7) -> (-9.18, -175.7)
  line L399 (-9.18, -175.7) -> (-9.18, -176.7)
  line L400 (-10.18, -175.7) -> (-27.88, -175.7)
  line L401 (-27.88, -175.7) -> (-27.88, -158)
  line L402 (-27.88, -158) -> (-10.18, -158)
  line L403 (-10.18, -158) -> (-10.18, -175.7)
  line L404 (8.52, -175.7) -> (-9.68, -175.7)
  line L405 (-9.68, -175.7) -> (-9.68, -158)
  line L406 (-9.68, -158) -> (8.52, -158)
  line L407 (8.52, -158) -> (8.52, -175.7)
  line L408 (-9.18, -250.5) -> (-10.18, -250.5)
  line L409 (-10.18, -250.5) -> (-10.18, -251.5)
  line L410 (-10.18, -251.5) -> (-9.18, -251.5)
  line L411 (-9.18, -251.5) -> (-9.18, -250.5)
  line L412 (-10.18, -251.5) -> (-27.88, -251.5)
  line L413 (-27.88, -251.5) -> (-27.88, -269.2)
  line L414 (-27.88, -269.2) -> (-10.18, -269.2)
  line L415 (-10.18, -269.2) -> (-10.18, -251.5)
  line L416 (-9.18, -213.1) -> (-10.18, -213.1)
  line L417 (-10.18, -213.1) -> (-10.18, -214.1)
  line L418 (-10.18, -214.1) -> (-9.18, -214.1)
  line L419 (-9.18, -214.1) -> (-9.18, -213.1)
  line L420 (-10.18, -214.1) -> (-27.88, -214.1)
  line L421 (-27.88, -214.1) -> (-27.88, -231.8)
  line L422 (-27.88, -231.8) -> (-10.18, -231.8)
  line L423 (-10.18, -231.8) -> (-10.18, -214.1)
  line L424 (-27.88, -231.8) -> (-28.88, -231.8)
  line L425 (-28.88, -231.8) -> (-28.88, -232.8)
  line L426 (-28.88, -232.8) -> (-27.88, -232.8)
  line L427 (-27.88, -232.8) -> (-27.88, -231.8)
  line L428 (-27.88, -232.8) -> (-10.18, -232.8)
  line L429 (-10.18, -232.8) -> (-10.18, -250.5)
  line L430 (-10.18, -250.5) -> (-27.88, -250.5)
  line L431 (-27.88, -250.5) -> (-27.88, -232.8)
  line L432 (-28.88, -232.8) -> (-46.58, -232.8)
  line L433 (-46.58, -232.8) -> (-46.58, -250.5)
  line L434 (-46.58, -250.5) -> (-28.88, -250.5)
  line L435 (-28.88, -250.5) -> (-28.88, -232.8)
  line L436 (-27.88, -214.1) -> (-28.88, -214.1)
  line L437 (-28.88, -214.1) -> (-28.88, -213.1)
  line L438 (-28.88, -213.1) -> (-27.88, -213.1)
  line L439 (-27.88, -213.1) -> (-27.88, -214.1)
  line L440 (-28.88, -213.1) -> (-46.58, -213.1)
  line L441 (-46.58, -213.1) -> (-46.58, -195.4)
  line L442 (-46.58, -195.4) -> (-28.88, -195.4)
  line L443 (-28.88, -195.4) -> (-28.88, -213.1)
  line L444 (-28.88, -195.4) -> (-27.88, -195.4)
  line L445 (-27.88, -195.4) -> (-27.88, -194.4)
  line L446 (-27.88, -194.4) -> (-28.88, -194.4)
  line L447 (-28.88, -194.4) -> (-28.88, -195.4)
  line L448 (-27.88, -194.4) -> (-10.18, -194.4)
  line L449 (-10.18, -194.4) -> (-10.18, -176.7)
  line L450 (-10.18, -176.7) -> (-27.88, -176.7)
  line L451 (-27.88, -176.7) -> (-27.88, -194.4)
  line L452 (-28.88, -194.4) -> (-46.58, -194.4)
  line L453 (-46.58, -194.4) -> (-46.58, -176.7)
  line L454 (-46.58, -176.7) -> (-28.88, -176.7)
  line L455 (-28.88, -176.7) -> (-28.88, -194.4)
  line L456 (-27.88, -195.4) -> (-10.18, -195.4)
  line L457 (-10.18, -195.4) -> (-10.18, -213.1)
  line L458 (-10.18, -213.1) -> (-27.88, -213.1)
  line L459 (-27.88, -213.1) -> (-27.88, -195.4)
  line L460 (-28.88, -214.1) -> (-46.58, -214.1)
  line L461 (-46.58, -214.1) -> (-46.58, -231.8)
  line L462 (-46.58, -231.8) -> (-28.88, -231.8)
  line L463 (-28.88, -231.8) -> (-28.88, -214.1)
  line L464 (9.52, -250.5) -> (27.22, -250.5)
  line L465 (27.22, -250.5) -> (27.22, -232.8)
  line L466 (27.22, -232.8) -> (9.52, -232.8)
  line L467 (9.52, -232.8) -> (9.52, -250.5)
  line L468 (9.52, -195.4) -> (27.22, -195.4)
  line L469 (27.22, -195.4) -> (27.22, -213.1)
  line L470 (27.22, -213.1) -> (9.52, -213.1)
  line L471 (9.52, -213.1) -> (9.52, -195.4)
  line L472 (8.52, -231.8) -> (-9.18, -231.8)
  line L473 (-9.18, -231.8) -> (-9.18, -214.1)
  line L474 (-9.18, -214.1) -> (8.52, -214.1)
  line L475 (8.52, -214.1) -> (8.52, -231.8)
  line L476 (8.52, -251.5) -> (-9.18, -251.5)
  line L477 (-9.18, -251.5) -> (-9.18, -269.2)
  line L478 (-9.18, -269.2) -> (8.52, -269.2)
  line L479 (8.52, -269.2) -> (8.52, -251.5)
  line L480 (33.42, -158) -> (27.22, -148)
  dimension "d86" = 6.2
  dimension "d87" = 10
  dimension "d88" = 73.8
  dimension "d89" = 111.2
  dimension "d90" = 17.7
  dimension "d91" = 17.7
  dimension "d92" = 17.7
  dimension "d93" = 17.7
  dimension "d94" = 17.7
  dimension "d95" = 17.7
  dimension "d96" = 17.7
  dimension "d97" = 17.7
  dimension "d98" = 1
  dimension "d99" = 1
  dimension "d100" = 17.7
  dimension "d101" = 17.7
  dimension "d102" = 1
  dimension "d103" = 1
  dimension "d104" = 17.7
  dimension "d105" = 17.7
  dimension "d106" = 1
  dimension "d107" = 1
  dimension "d108" = 17.7
  dimension "d109" = 17.7
  dimension "d110" = 1
  dimension "d111" = 1
  dimension "d112" = 17.7
  dimension "d113" = 17.7
  dimension "d114" = 1
  dimension "d115" = 1
  dimension "d116" = 17.7
  dimension "d117" = 17.7
  dimension "d118" = 1
  dimension "d119" = 1
  dimension "d120" = 17.7
  dimension "d121" = 17.7
  dimension "d122" = 1
  dimension "d123" = 1
  dimension "d124" = 17.7
  dimension "d125" = 17.7
  dimension "d126" = 1
  dimension "d127" = 1
  dimension "d128" = 17.7
  dimension "d129" = 17.7
  dimension "d130" = 1
  dimension "d131" = 1
  dimension "d132" = 17.7
  dimension "d133" = 1
  dimension "d134" = 1
  dimension "d135" = 17.7
  dimension "d136" = 1
  dimension "d137" = 1
  dimension "d138" = 17.7
  dimension "d139" = 17.7
  dimension "d140" = 17.7
  constraint horizontal L328
  constraint vertical L329
  constraint horizontal L330
  constraint vertical L331
  constraint coincident L241.end L242.start
  constraint coincident L307.end L308.start
  constraint horizontal L332
  constraint vertical L333
  constraint horizontal L334
  constraint vertical L335
  constraint horizontal L336
  constraint vertical L337
  constraint horizontal L338
  constraint vertical L339
  constraint horizontal L340
  constraint vertical L341
  constraint horizontal L342
  constraint vertical L343
  constraint horizontal L344
  constraint vertical L345
  constraint horizontal L346
  constraint vertical L347
  constraint horizontal L348
  constraint vertical L349
  constraint horizontal L350
  constraint vertical L351
  constraint horizontal L352
  constraint vertical L353
  constraint horizontal L354
  constraint vertical L355
  constraint horizontal L356
  constraint vertical L357
  constraint horizontal L358
  constraint vertical L359
  constraint horizontal L360
  constraint vertical L361
  constraint horizontal L362
  constraint vertical L363
  constraint horizontal L364
  constraint vertical L365
  constraint horizontal L366
  constraint vertical L367
  constraint horizontal L368
  constraint vertical L369
  constraint horizontal L370
  constraint vertical L371
  constraint horizontal L372
  constraint vertical L373
  constraint horizontal L374
  constraint vertical L375
  constraint horizontal L376
  constraint vertical L377
  constraint horizontal L378
  constraint vertical L379
  constraint horizontal L380
  constraint vertical L381
  constraint horizontal L382
  constraint vertical L383
  constraint horizontal L384
  constraint vertical L385
  constraint horizontal L386
  constraint vertical L387
  constraint horizontal L388
  constraint vertical L389
  constraint horizontal L390
  constraint vertical L391
  constraint horizontal L392
  constraint vertical L393
  constraint horizontal L394
  constraint vertical L395
  constraint horizontal L396
  constraint vertical L397
  constraint horizontal L398
  constraint vertical L399
  constraint horizontal L400
  constraint vertical L401
  constraint horizontal L402
  constraint vertical L403
  constraint horizontal L404
  constraint vertical L405
  constraint horizontal L406
  constraint vertical L407
  constraint midpoint L336 L405.end
  constraint horizontal L408
  constraint vertical L409
  constraint horizontal L410
  constraint vertical L411
  constraint horizontal L412
  constraint vertical L413
  constraint horizontal L414
  constraint vertical L415
  constraint horizontal L416
  constraint vertical L417
  constraint horizontal L418
  constraint vertical L419
  constraint horizontal L420
  constraint vertical L421
  constraint horizontal L422
  constraint vertical L423
  constraint horizontal L424
  constraint vertical L425
  constraint horizontal L426
  constraint vertical L427
  constraint horizontal L428
  constraint vertical L429
  constraint horizontal L430
  constraint vertical L431
  constraint horizontal L432
  constraint vertical L433
  constraint horizontal L434
  constraint vertical L435
  constraint coincident L337 L433.end
  constraint horizontal L436
  constraint vertical L437
  constraint horizontal L438
  constraint vertical L439
  constraint horizontal L440
  constraint vertical L441
  constraint horizontal L442
  constraint vertical L443
  constraint horizontal L444
  constraint vertical L445
  constraint horizontal L446
  constraint vertical L447
  constraint horizontal L448
  constraint vertical L449
  constraint horizontal L450
  constraint vertical L451
  constraint horizontal L452
  constraint vertical L453
  constraint horizontal L454
  constraint vertical L455
  constraint horizontal L456
  constraint vertical L457
  constraint horizontal L458
  constraint vertical L459
  constraint horizontal L460
  constraint vertical L461
  constraint horizontal L462
  constraint vertical L463
  constraint horizontal L464
  constraint vertical L465
  constraint horizontal L466
  constraint vertical L467
  constraint coincident L339 L465.end
  constraint horizontal L468
  constraint vertical L469
  constraint horizontal L470
  constraint vertical L471
  constraint coincident L339 L469.end
  constraint horizontal L472
  constraint vertical L473
  constraint horizontal L474
  constraint vertical L475
  constraint horizontal L476
  constraint vertical L477
  constraint horizontal L478
  constraint vertical L479
  constraint coincident L338 L477.end
  measures "d86" distance of L299.end L332.end
  measures "d87" distance of L299.end L334.end
  measures "d88" distance of L333.end L336.end
  measures "d89" distance of L333.end L338.end
  measures "d90" distance of L333.end L340.end
  measures "d91" distance of L333.end L342.end
  measures "d92" distance of L336.end L344.end
  measures "d93" distance of L336.end L346.end
  measures "d94" distance of L337.end L348.end
  measures "d95" distance of L337.end L350.end
  measures "d96" distance of L338.end L352.end
  measures "d97" distance of L338.end L354.end
  measures "d98" distance of L353.end L356.end
  measures "d99" distance of L353.end L358.end
  measures "d100" distance of L357.end L360.end
  measures "d101" distance of L357.end L362.end
  measures "d102" distance of L362.end L364.end
  measures "d103" distance of L362.end L366.end
  measures "d104" distance of L365.end L368.end
  measures "d105" distance of L365.end L370.end
  measures "d106" distance of L370.end L372.end
  measures "d107" distance of L370.end L374.end
  measures "d108" distance of L373.end L376.end
  measures "d109" distance of L373.end L378.end
  measures "d110" distance of L378.end L380.end
  measures "d111" distance of L378.end L382.end
  measures "d112" distance of L381.end L384.end
  measures "d113" distance of L381.end L386.end
  measures "d114" distance of L341.end L388.end
  measures "d115" distance of L341.end L386.end
  measures "d116" distance of L389.end L392.end
  measures "d117" distance of L389.end L382.end